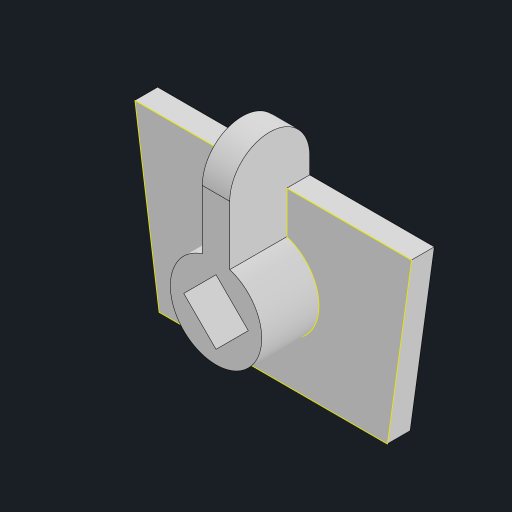
# Autodesk Inventor part: om_BackHolder_V3
Saved by Autodesk Inventor 2023 (Build 270158000, 158)
## iProperties
Created: 2022-07-14
Part Number: om_BackHolder_V3
Material: 一般
Document SubType Name: Modeling
Designer: legot
Density: 1 g/cm^3
Appearance: 既定
Author: legot
Autodesk Inventor part; units mm, degrees
ref_plane "YZ Plane" through (0, 0, 0) normal (1, 0, 0) x (0, 1, 0)
ref_plane "XZ Plane" through (0, 0, 0) normal (0, 1, 0) x (-1, 0, 0)
ref_plane "XY Plane" through (0, 0, 0) normal (0, 0, 1) x (1, 0, 0)
sketch "スケッチ1" plane through (0, 0, 0) normal (0, 0, 1) x (1, 0, 0)
  line L0 (2.8284, 0) -> (0, -2.8284)
  line L1 (0, -2.8284) -> (-2.8284, 0)
  line L2 (-2.8284, 0) -> (0, 2.8284)
  line L3 (0, 2.8284) -> (2.8284, 0)
  line L4 (-12.1149, 7.5) -> (-10, -7.5)
  line L5 (10, -7.5) -> (-10, -7.5)
  line L6 (10, -7.5) -> (12.1149, 7.5)
  line L7 (12.1149, 7.5) -> (-12.1149, 7.5)
  point P0 (0, 0)
  point P1 (0, 7.5)
  point P2 (11.0574, 0)
  dimension "d10" = 24.2298
  dimension "d11" = 20
  dimension "d12" = 15
  dimension "d13" = 4
  constraints: 16 end point, 4 equal length, 3 vertical alignment, 2 horizontal alignment, 2 midpoint, 1 horizontal, 1 perpendicular
  measures "d10" distance of L6.end L4.start
  measures "d11" distance of L5.start L4.end
  measures "d12" distance between parallel lines of L7 L5
  measures "d13" distance of L2.end L0.start
extrude "押し出し1" add sketch "スケッチ1" against normal blind 2
sketch "スケッチ3" plane through (0, 0, 0) normal (0, 0, 1) x (1, 0, 0)
  line L0 (2.8284, 0) -> (0, -2.8284) projected
  line L1 (0, -2.8284) -> (-2.8284, 0) projected
  line L2 (-2.8284, 0) -> (0, 2.8284) projected
  line L3 (0, 2.8284) -> (2.8284, 0) projected
  circle A0 centre (0, 0) radius 4
  dimension "d17" = 8
  constraints: 1 centre point, 1 coincident
  measures "d17" diameter of A0
extrude "押し出し3" add sketch "スケッチ3" along normal blind 5
sketch "スケッチ4" plane through (0, 0, 5) normal (0, 0, 1) x (1, 0, 0)
  circle A0 centre (0, 0) radius 4 projected
  circle A1 centre (0, 0) radius 4 projected
  line L0 (-1.2, 3.8158) -> (-1.2, 12.5)
  line L1 (-1.2, 12.5) -> (1.2, 12.5)
  line L2 (1.2, 12.5) -> (1.2, 3.8158)
  line L3 (12.1149, 7.5) -> (-12.1149, 7.5) construction
  dimension "d18" = 5
  dimension "d19" = 2.4
  constraints: 6 end point, 2 perpendicular, 2 point on circle, 1 horizontal alignment, 1 vertical
  measures "d18" distance between parallel lines of L1 L3
  measures "d19" distance of L0.end L1.end
extrude "押し出し4" add sketch "スケッチ4" against normal up to surface (7 mm away) contours A0 L0 L1 L2
sketch "スケッチ5" plane through (1.2, 3.8158, 5) normal (1, 0, 0) x (0, 0, -1)
  line L0 (7, 3.6842) -> (7, 8.6842) projected
  line L1 (0, 8.6842) -> (7, 8.6842) projected
  line L2 (0, 0) -> (0, 8.6842) projected
  arc A0 (7, 5.1842) -> (0, 5.1842) centre (3.5, 5.1842) ccw
  point P0 (5, -3.8158)
  point P1 (3.5, 8.6842)
  constraints: 3 tangent, 2 point on circle, 2 point on line, 1 centre point
extrude "押し出し5" cut sketch "スケッチ5" along normal through all both and the other way through all
sketch "スケッチ7" plane through (0, 0, 0) normal (0, 0, 1) x (1, 0, 0)
  line L0 (-1.2, 3.8158) -> (-1.2, 7.5) projected
  line L1 (-1.2, 7.5) -> (-12.1149, 7.5) projected
  line L2 (-12.1149, 7.5) -> (-10, -7.5) projected
  line L3 (-10, -7.5) -> (10, -7.5) projected
  line L4 (10, -7.5) -> (12.1149, 7.5) projected
  line L5 (12.1149, 7.5) -> (1.2, 7.5) projected
  line L6 (1.2, 7.5) -> (1.2, 3.8158) projected
  arc A0 (-1.2, 3.8158) -> (1.2, 3.8158) centre (0, 0) ccw projected
